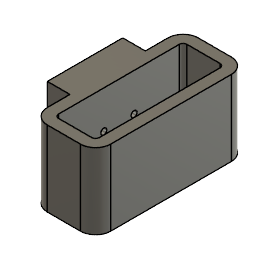
_Untitled.8da377d0-d6b8-4dad-80bb-bf51dc633e5f (Autodesk Fusion 360 design; units mm, degrees)
Autodesk Fusion 360 part; units mm, degrees
sketch "Sketch1" plane through (0, 0, 0) normal (1, 0, 0) x (0, 0, -1)
sketch "Sketch2" plane through (0, 0, 0) normal (0, 1, 0) x (1, 0, 0)
  line L0 (10, 0) -> (32, 0)
  line L1 (42, -10) -> (42, -90)
  line L2 (32, -100) -> (10, -100)
  line L3 (0, -25) -> (-15, -25)
  line L4 (-15, -25) -> (-15, -75)
  line L5 (-15, -75) -> (0, -75)
  arc A0 (10, 0) -> (0, -10) centre (10, -10) ccw
  arc A1 (42, -10) -> (32, 0) centre (32, -10) ccw
  arc A2 (32, -100) -> (42, -90) centre (32, -90) ccw
  arc A3 (0, -90) -> (10, -100) centre (10, -90) ccw
  arc A4 (10, -7.5) -> (7.5, -10) centre (10, -10) ccw
  line L6 (7.5, -90) -> (7.5, -10)
  arc A5 (7.5, -90) -> (10, -92.5) centre (10, -90) ccw
  line L7 (32, -92.5) -> (10, -92.5)
  arc A6 (32, -92.5) -> (34.5, -90) centre (32, -90) ccw
  line L8 (34.5, -10) -> (34.5, -90)
  arc A7 (34.5, -10) -> (32, -7.5) centre (32, -10) ccw
  line L9 (10, -7.5) -> (32, -7.5)
  line L10 (0, -90) -> (0, -75)
  line L11 (0, -25) -> (0, -10)
  point P0 (42, 0)
  point P1 (0, -100)
  dimension "d11" = 42
  constraint horizontal L0
  constraint vertical L1
  constraint horizontal L2
  constraint vertical L10
  constraint horizontal L3
  constraint vertical L4
  constraint horizontal L5
  constraint coincident L3.start L10
  constraint coincident origin L0
  constraint coincident origin L10
  constraint tangent L0 A0
  constraint tangent A0 L10
  constraint coincident P0 L0
  constraint coincident P0 L1
  constraint tangent L0 A1
  constraint tangent L1 A1
  constraint equal A0 A1
  constraint tangent L1 A2
  constraint tangent L2 A2
  constraint equal A0 A2
  constraint coincident P1 L2
  constraint coincident P1 L10
  constraint tangent L2 A3
  constraint tangent A3 L10
  constraint equal A0 A3
  constraint concentric A0 A4
  constraint concentric A3 A5
  constraint concentric A2 A6
  constraint concentric A1 A7
  constraint tangent A4 L9
  constraint tangent A7 L9
  constraint tangent L6 A5
  constraint tangent A4 L6
  constraint tangent L8 A7
  constraint tangent A5 L7
  constraint tangent L7 A6
  constraint tangent A6 L8
  constraint collinear L10 L11
  measures "d11" distance of L1 L11
extrude "Extrude1" add sketch "Sketch2" along normal blind 50
sketch "Sketch3" plane through (-15, 0, 0) normal (-1, 0, 0) x (0, 0, 1)
  line L0 (25, 0) -> (75, 0)
  line L1 (75, 0) -> (75, 50)
  line L2 (75, 50) -> (25, 50)
  line L3 (25, 50) -> (25, 0)
  circle A0 centre (40, 25) radius 2
  circle A1 centre (60, 25) radius 2
  dimension "d7" = 4
  dimension "d8" = 4
  measures "d7" diameter of A0
  measures "d8" diameter of A1
extrude "Extrude2" cut sketch "Sketch3" against normal blind 45 contours A0 | A1
